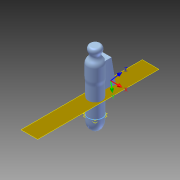
# Autodesk Inventor part: Handle_1_backup
Saved by Autodesk Inventor 2011 SP2 (Build 150309200, 309)
## iProperties
Created: 2012-02-26
Part Number: Handle_1_backup
Document SubType Name: Modeling
Designer: sungwook
Density: 1 g/cm^3
Author: sungwook
Autodesk Inventor part; units mm, degrees
note: some values were not read from the file. Chosen so that the rebuilt part matches the saved one: direction of "Hole2".
(part 1 of 18)
ref_plane "YZ Plane" through (0, 0, 0) normal (1, 0, 0) x (0, 1, 0)
sketch "Handle_0" plane through (0, 0, 0) normal (0, 0, 1) x (1, 0, 0)
  spline S0 degree 3 poles (-10017.4276, -10030.2974) (-10017.014, -10030.1564) (-10016.1737, -10029.8699) (-10014.8677, -10029.4935) (-10013.4915, -10029.1726) (-10012.0789, -10028.9345) (-10010.6777, -10028.7846) (-10009.3294, -10028.7092) (-10008.027, -10028.6839) (-10007.1723, -10028.6839) (-10006.75, -10028.6838) knots 0 0 0 0 0.131107 0.266278 0.407581 0.554823 0.69573 0.830104 0.959816 1.086502 1.086502 1.086502 1.086502
  spline S1 degree 3 poles (-10021.7321, -10032.2974) (-10021.7323, -10032.2974) (-10021.7332, -10032.2974) (-10021.7351, -10032.2974) (-10021.7383, -10032.2974) (-10021.7427, -10032.2974) (-10021.7484, -10032.2974) (-10021.7553, -10032.2974) (-10021.7635, -10032.2974) (-10021.7729, -10032.2974) (-10021.7836, -10032.2974) (-10021.7954, -10032.2974) (-10021.8085, -10032.2974) (-10021.8228, -10032.2974) (-10021.8383, -10032.2974) (-10021.8549, -10032.2974) (-10021.8727, -10032.2974) (-10021.8849, -10032.2974) (-10021.8912, -10032.2974) knots 0 0 0 0 0.003987 0.015957 0.035891 0.063749 0.099497 0.143102 0.194528 0.253743 0.320712 0.395401 0.477746 0.567575 0.664794 0.769325 0.881087 1 1 1 1
  spline S2 degree 3 poles (-10021.8912, -10032.2974) (-10021.5076, -10032.1439) (-10020.7463, -10031.8393) (-10019.2614, -10031.1643) (-10018.1607, -10030.6439) (-10017.4276, -10030.2974) knots 0 0 0 0 0.253343 0.502767 1 1 1 1
  spline S3 degree 3 poles (-10017.7909, -10013.9834) (-10017.3644, -10014.133) (-10016.4972, -10014.4372) (-10015.1487, -10014.8433) (-10013.7243, -10015.1928) (-10012.2605, -10015.4542) (-10010.8089, -10015.6192) (-10009.4142, -10015.7024) (-10008.0687, -10015.7302) (-10007.1861, -10015.7302) (-10006.75, -10015.7303) knots 0 0 0 0 0.135587 0.27568 0.422315 0.575323 0.72143 0.860365 0.994299 1.125132 1.125132 1.125132 1.125132
  line L0 (-10022.3039, -10015.9834) -> (-10006.75, -10015.9834)
  line L1 (-10006.75, -10015.7303) -> (-10006.75, -10015.9834)
  line L2 (-10006.75, -10015.9834) -> (-10006.75, -10017.9834)
  spline S4 degree 3 poles (-10006.75, -10017.9834) (-10007.6323, -10017.9834) (-10008.9768, -10017.9834) (-10010.805, -10017.9834) (-10012.253, -10017.9834) (-10013.7139, -10017.9834) (-10015.1384, -10017.9834) (-10016.4885, -10017.9834) (-10017.3635, -10017.9834) (-10017.7912, -10017.9834) knots 0 0 0 0 0.264693 0.403339 0.548464 0.699098 0.841605 0.975818 1.104119 1.104119 1.104119 1.104119
  spline S5 degree 3 poles (-10017.7912, -10017.9834) (-10018.5274, -10017.6306) (-10019.6344, -10017.1002) (-10020.9473, -10016.5195) (-10021.7151, -10016.205) (-10022.1069, -10016.0575) (-10022.3039, -10015.9834) knots 0 0 0 0 0.495968 0.745691 0.872094 1 1 1 1
  spline S6 degree 3 poles (-10022.3039, -10015.9834) (-10022.2789, -10015.9018) (-10022.229, -10015.7391) (-10022.1784, -10015.4891) (-10022.1468, -10015.237) (-10022.1364, -10014.9833) (-10022.1468, -10014.7297) (-10022.1783, -10014.4775) (-10022.2289, -10014.2276) (-10022.2788, -10014.0649) (-10022.3038, -10013.9834) knots 0 0 0 0 0.125726 0.250746 0.375528 0.500005 0.624584 0.749245 0.874433 1 1 1 1
  spline S7 degree 3 poles (-10022.3038, -10013.9834) (-10021.9144, -10013.9834) (-10021.1487, -10013.9834) (-10019.6444, -10013.9834) (-10018.5295, -10013.9834) (-10017.7909, -10013.9834) knots 0 0 0 0 0.25882 0.509015 1 1 1 1
  line L3 (-10033.25, -10030.2974) -> (-10017.4276, -10030.2974)
  line L4 (-10033.25, -10030.2974) -> (-10033.25, -10028.2974)
  line L5 (-10033.25, -10028.2974) -> (-10006.75, -10028.2974)
  line L6 (-10033.25, -10032.2974) -> (-10021.8912, -10032.2974)
  line L7 (-10033.25, -10032.2974) -> (-10033.25, -10030.2974)
  line L8 (-10033.25, -10017.9834) -> (-10017.7912, -10017.9834)
  line L9 (-10033.25, -10017.9834) -> (-10033.25, -10015.9834)
  line L10 (-10033.25, -10015.9834) -> (-10022.3039, -10015.9834)
  line L11 (-10033.25, -10015.9834) -> (-10033.25, -10013.9834)
  line L12 (-10033.25, -10013.9834) -> (-10022.3038, -10013.9834)
  line L13 (-10033.25, -10018.7294) -> (-10006.75, -10018.7294)
  line L14 (-10033.25, -10018.7294) -> (-10033.25, -10017.9834)
  line L15 (-10033.25, -10016.7294) -> (-10006.75, -10016.7294)
  line L16 (-10033.25, -10014.7294) -> (-10017.2831, -10014.7294)
  spline S8 degree 3 poles (-10006.75, -10016.3506) (-10007.1666, -10016.3506) (-10008.0095, -10016.3506) (-10009.294, -10016.3252) (-10010.6236, -10016.2493) (-10012.0057, -10016.0986) (-10013.3997, -10015.8592) (-10014.758, -10015.5367) (-10016.0468, -10015.1587) (-10016.8753, -10014.871) (-10017.2831, -10014.7294) knots 0 0 0 0 0.124973 0.252876 0.385371 0.524366 0.669742 0.809378 0.942972 1.072465 1.072465 1.072465 1.072465
  spline S9 degree 3 poles (-10022.0472, -10014.7294) (-10022.0417, -10014.8155) (-10022.0307, -10014.9878) (-10022.0416, -10015.2468) (-10022.0725, -10015.5043) (-10022.1248, -10015.7593) (-10022.1972, -10016.0104) (-10022.2891, -10016.2566) (-10022.398, -10016.4976) (-10022.4841, -10016.652) (-10022.5273, -10016.7294) knots 0 0 0 0 0.12386 0.247576 0.371585 0.495852 0.620749 0.746432 0.87277 1 1 1 1
  spline S10 degree 3 poles (-10022.5273, -10016.7294) (-10022.3413, -10016.8015) (-10021.9712, -10016.9449) (-10021.2455, -10017.2527) (-10020.357, -10017.6621) (-10019.3096, -10018.1858) (-10018.6193, -10018.548) (-10018.2736, -10018.7294) knots 0 0 0 0 0.127199 0.253182 0.502754 0.751027 1 1 1 1
  line L17 (-10035.75, -10008.8034) -> (-10035.75, -10032.8034)
  line L18 (-10149.7109, -10011.3194) -> (-10149.7109, -10030.2874)
  line L19 (-10149.3255, -10010.8327) -> (-10149.3255, -10030.7741)
  spline S11 degree 3 poles (-10130.7269, -10031.7874) (-10130.926, -10031.6416) (-10131.3276, -10031.3477) (-10132.101, -10030.7002) (-10132.8603, -10030.0211) (-10133.6568, -10029.3749) (-10134.1857, -10029.0056) (-10134.6323, -10028.7443) (-10134.9822, -10028.5682) (-10135.3467, -10028.4119) (-10135.5994, -10028.3291) (-10135.7269, -10028.2874) knots 0 0 0 0 0.074013 0.149267 0.302447 0.379596 0.456855 0.495662 0.534746 0.574288 0.614507 0.614507 0.614507 0.614507
  spline S12 degree 3 poles (-10130.7269, -10009.8194) (-10130.926, -10009.9651) (-10131.3276, -10010.2591) (-10132.101, -10010.9066) (-10132.8603, -10011.5857) (-10133.6568, -10012.2319) (-10134.1857, -10012.6012) (-10134.6323, -10012.8625) (-10134.9822, -10013.0385) (-10135.3467, -10013.1949) (-10135.5994, -10013.2777) (-10135.7269, -10013.3194) knots 0 0 0 0 0.074013 0.149267 0.302447 0.379596 0.456855 0.495662 0.534746 0.574288 0.614507 0.614507 0.614507 0.614507
  spline S13 degree 3 poles (-10125.7269, -10033.3034) (-10125.9497, -10033.3002) (-10126.3951, -10033.294) (-10127.0596, -10033.2345) (-10127.7155, -10033.1289) (-10128.3575, -10032.9694) (-10128.9818, -10032.7548) (-10129.5857, -10032.4841) (-10130.1707, -10032.1631) (-10130.5407, -10031.9132) (-10130.7269, -10031.7874) knots 0 0 0 0 0.066832 0.133581 0.19996 0.265954 0.331772 0.397749 0.464268 0.531651 0.531651 0.531651 0.531651
  spline S14 degree 3 poles (-10125.7269, -10008.3034) (-10125.9497, -10008.3065) (-10126.3951, -10008.3128) (-10127.0596, -10008.3723) (-10127.7155, -10008.4778) (-10128.3575, -10008.6374) (-10128.9818, -10008.8519) (-10129.5857, -10009.1227) (-10130.1707, -10009.4437) (-10130.5407, -10009.6936) (-10130.7269, -10009.8194) knots 0 0 0 0 0.066832 0.133581 0.19996 0.265954 0.331772 0.397749 0.464268 0.531651 0.531651 0.531651 0.531651
  arc A0 (-10149.3255, -10010.8327) -> (-10149.7109, -10011.3194) centre (-10149.2109, -10011.3194) ccw
  arc A1 (-10149.7109, -10030.2874) -> (-10149.3255, -10030.7741) centre (-10149.2109, -10030.2874) ccw
  spline S15 degree 3 poles (-10135.7269, -10028.2874) (-10135.9278, -10028.2333) (-10136.3389, -10028.1224) (-10136.9908, -10028.0381) (-10137.6833, -10028.0106) (-10138.4185, -10028.0482) (-10139.195, -10028.1445) (-10140.0117, -10028.2962) (-10140.8656, -10028.4992) (-10142.0718, -10028.8328) (-10143.63, -10029.3289) (-10145.5262, -10029.9531) (-10147.1288, -10030.4125) (-10148.3979, -10030.6807) (-10149.0212, -10030.7434) (-10149.3255, -10030.7741) knots 0 0 0 0 0.062347 0.127633 0.196641 0.270049 0.348203 0.431234 0.519115 0.611423 0.806629 1.009594 1.210352 1.306485 1.398176 1.398176 1.398176 1.398176
  spline S16 degree 3 poles (-10135.7269, -10013.3194) (-10135.9278, -10013.3735) (-10136.3389, -10013.4843) (-10136.9908, -10013.5687) (-10137.6833, -10013.5961) (-10138.4185, -10013.5586) (-10139.195, -10013.4622) (-10140.0117, -10013.3105) (-10140.8656, -10013.1076) (-10142.0718, -10012.774) (-10143.63, -10012.2779) (-10145.5262, -10011.6537) (-10147.1288, -10011.1943) (-10148.3979, -10010.9261) (-10149.0212, -10010.8633) (-10149.3255, -10010.8327) knots 0 0 0 0 0.062347 0.127633 0.196641 0.270049 0.348203 0.431234 0.519115 0.611423 0.806629 1.009594 1.210352 1.306485 1.398176 1.398176 1.398176 1.398176
  line L20 (-10150.7269, -10009.8034) -> (-10150.7269, -10031.8034)
  spline S17 degree 3 poles (-10135.7269, -10029.3034) (-10135.5108, -10029.4039) (-10135.0741, -10029.6072) (-10134.4442, -10029.9821) (-10133.8129, -10030.3902) (-10133.18, -10030.8311) (-10132.5504, -10031.3008) (-10131.7333, -10031.962) (-10131.1285, -10032.4676) (-10130.7269, -10032.8034) knots 0 0 0 0 0.071451 0.144434 0.219638 0.296973 0.375788 0.45523 0.612272 0.612272 0.612272 0.612272
  spline S18 degree 3 poles (-10135.7269, -10012.3034) (-10135.5108, -10012.2028) (-10135.0741, -10011.9996) (-10134.4442, -10011.6247) (-10133.8129, -10011.2166) (-10133.18, -10010.7757) (-10132.5504, -10010.306) (-10131.7333, -10009.6447) (-10131.1285, -10009.1391) (-10130.7269, -10008.8034) knots 0 0 0 0 0.071451 0.144434 0.219638 0.296973 0.375788 0.45523 0.612272 0.612272 0.612272 0.612272
  spline S19 degree 3 poles (-10130.7269, -10032.8034) (-10130.5423, -10032.9469) (-10130.2674, -10033.1606) (-10129.884, -10033.4163) (-10129.594, -10033.5901) (-10129.2985, -10033.7456) (-10128.9973, -10033.882) (-10128.6898, -10033.9984) (-10128.3763, -10034.0947) (-10128.0571, -10034.172) (-10127.6231, -10034.2505) (-10127.0692, -10034.306) (-10126.3992, -10034.3225) (-10125.9509, -10034.3204) (-10125.7269, -10034.3194) knots 0 0 0 0 0.070131 0.104405 0.138173 0.17151 0.20452 0.237328 0.270066 0.302853 0.33579 0.402309 0.469592 0.53679 0.53679 0.53679 0.53679
  spline S20 degree 3 poles (-10130.7269, -10008.8034) (-10130.5423, -10008.6598) (-10130.2674, -10008.4461) (-10129.884, -10008.1905) (-10129.594, -10008.0167) (-10129.2985, -10007.8612) (-10128.9973, -10007.7247) (-10128.6898, -10007.6084) (-10128.3763, -10007.5121) (-10128.0571, -10007.4348) (-10127.6231, -10007.3563) (-10127.0692, -10007.3007) (-10126.3992, -10007.2843) (-10125.9509, -10007.2864) (-10125.7269, -10007.2874) knots 0 0 0 0 0.070131 0.104405 0.138173 0.17151 0.20452 0.237328 0.270066 0.302853 0.33579 0.402309 0.469592 0.53679 0.53679 0.53679 0.53679
  spline S21 degree 3 poles (-10149.7109, -10031.8034) (-10149.3939, -10031.7865) (-10148.7265, -10031.7511) (-10147.7049, -10031.5383) (-10146.6313, -10031.2587) (-10145.1692, -10030.808) (-10143.7277, -10030.3152) (-10142.32, -10029.8454) (-10141.3329, -10029.5329) (-10140.407, -10029.2713) (-10139.5489, -10029.0697) (-10138.761, -10028.9335) (-10138.0418, -10028.87) (-10137.3871, -10028.8799) (-10136.7899, -10028.9587) (-10136.2385, -10029.099) (-10135.8958, -10029.2359) (-10135.7269, -10029.3034) knots 0 0 0 0 0.095122 0.200216 0.312183 0.428034 0.659064 0.769198 0.873257 0.96964 1.057768 1.137592 1.209313 1.274064 1.333591 1.389675 1.444205 1.444205 1.444205 1.444205
  spline S22 degree 3 poles (-10149.7109, -10009.8034) (-10149.3939, -10009.8202) (-10148.7265, -10009.8557) (-10147.7049, -10010.0685) (-10146.6313, -10010.3481) (-10145.1692, -10010.7988) (-10143.7277, -10011.2916) (-10142.32, -10011.7614) (-10141.3329, -10012.0739) (-10140.407, -10012.3355) (-10139.5489, -10012.5371) (-10138.761, -10012.6733) (-10138.0418, -10012.7368) (-10137.3871, -10012.7269) (-10136.7899, -10012.6481) (-10136.2385, -10012.5077) (-10135.8958, -10012.3709) (-10135.7269, -10012.3034) knots 0 0 0 0 0.095122 0.200216 0.312183 0.428034 0.659064 0.769198 0.873257 0.96964 1.057768 1.137592 1.209313 1.274064 1.333591 1.389675 1.444205 1.444205 1.444205 1.444205
  line L21 (-10149.7109, -10031.8034) -> (-10150.7269, -10031.8034)
  line L22 (-10149.7109, -10009.8034) -> (-10150.7269, -10009.8034)
  line L23 (-10006.75, -10012.8034) -> (-10006.75, -10015.7303)
  line L24 (-10006.75, -10017.9834) -> (-10006.75, -10028.6838)
  spline S23 degree 3 poles (-10031.75, -10033.8194) (-10030.8977, -10033.8186) (-10029.6216, -10033.8174) (-10027.9256, -10033.7166) (-10026.664, -10033.5781) (-10025.4125, -10033.368) (-10024.1727, -10033.0817) (-10022.9433, -10032.7265) (-10022.1369, -10032.4408) (-10021.7321, -10032.2974) knots 0 0 0 0 0.25561 0.382747 0.509496 0.636178 0.763224 0.891032 1.019834 1.019834 1.019834 1.019834
  spline S24 degree 3 poles (-10031.75, -10007.7874) (-10030.68, -10007.7919) (-10029.0783, -10007.7987) (-10026.9528, -10007.9822) (-10025.3776, -10008.2408) (-10023.8213, -10008.6177) (-10021.7597, -10009.2599) (-10019.25, -10010.2954) (-10016.7403, -10011.3308) (-10014.6787, -10011.973) (-10013.1224, -10012.35) (-10011.5472, -10012.6085) (-10009.4217, -10012.792) (-10007.82, -10012.7988) (-10006.75, -10012.8034) knots 0 0 0 0 0.320849 0.480281 0.639462 0.799243 0.960292 1.286737 1.613182 1.774231 1.934012 2.093192 2.252625 2.573474 2.573474 2.573474 2.573474
  line L25 (-10035.75, -10015.8034) -> (-10006.75, -10015.8034)
  line L26 (-10035.75, -10025.8034) -> (-10006.75, -10025.8034)
  line L27 (-10035.75, -10015.8404) -> (-10033.25, -10015.8404)
  line L28 (-10035.75, -10017.6184) -> (-10033.25, -10017.6184)
  line L29 (-10035.75, -10015.0944) -> (-10033.25, -10015.0944)
  line L30 (-10035.75, -10016.8724) -> (-10033.25, -10016.8724)
  line L31 (-10035.75, -10029.4084) -> (-10033.25, -10029.4084)
  line L32 (-10035.75, -10031.1864) -> (-10033.25, -10031.1864)
  line L33 (-10035.75, -10032.8034) -> (-10095.75, -10032.8034)
  line L34 (-10035.75, -10008.8034) -> (-10095.75, -10008.8034)
  line L35 (-10031.75, -10033.8194) -> (-10095.75, -10033.8194)
  line L36 (-10031.75, -10007.7874) -> (-10095.75, -10007.7874)
  spline S25 degree 3 poles (-10095.75, -10032.8034) (-10095.9588, -10032.8037) (-10096.376, -10032.8044) (-10097.0013, -10032.8424) (-10097.6226, -10032.9293) (-10098.2385, -10033.0534) (-10098.8543, -10033.1775) (-10099.4756, -10033.2644) (-10100.1009, -10033.3024) (-10100.5181, -10033.303) (-10100.7269, -10033.3034) knots 0 0 0 0 0.062631 0.12514 0.187761 0.250672 0.313584 0.376205 0.438713 0.501345 0.501345 0.501345 0.501345
  spline S26 degree 3 poles (-10095.75, -10008.8034) (-10095.9588, -10008.803) (-10096.376, -10008.8024) (-10097.0013, -10008.7644) (-10097.6226, -10008.6775) (-10098.2385, -10008.5534) (-10098.8543, -10008.4293) (-10099.4756, -10008.3424) (-10100.1009, -10008.3044) (-10100.5181, -10008.3037) (-10100.7269, -10008.3034) knots 0 0 0 0 0.062631 0.12514 0.187761 0.250672 0.313584 0.376205 0.438713 0.501345 0.501345 0.501345 0.501345
  spline S27 degree 3 poles (-10100.7269, -10034.3194) (-10100.5181, -10034.319) (-10100.1009, -10034.3184) (-10099.4756, -10034.2804) (-10098.8543, -10034.1935) (-10098.2385, -10034.0694) (-10097.6226, -10033.9453) (-10097.0013, -10033.8584) (-10096.376, -10033.8204) (-10095.9588, -10033.8197) (-10095.75, -10033.8194) knots 0 0 0 0 0.062631 0.12514 0.187761 0.250672 0.313584 0.376205 0.438713 0.501345 0.501345 0.501345 0.501345
  spline S28 degree 3 poles (-10100.7269, -10007.2874) (-10100.5181, -10007.2877) (-10100.1009, -10007.2884) (-10099.4756, -10007.3264) (-10098.8543, -10007.4133) (-10098.2385, -10007.5374) (-10097.6226, -10007.6615) (-10097.0013, -10007.7484) (-10096.376, -10007.7864) (-10095.9588, -10007.787) (-10095.75, -10007.7874) knots 0 0 0 0 0.062631 0.12514 0.187761 0.250672 0.313584 0.376205 0.438713 0.501345 0.501345 0.501345 0.501345
  line L37 (-10100.7269, -10033.3034) -> (-10125.7269, -10033.3034)
  line L38 (-10100.7269, -10008.3034) -> (-10125.7269, -10008.3034)
  line L39 (-10100.7269, -10034.3194) -> (-10125.7269, -10034.3194)
  line L40 (-10100.7269, -10007.2874) -> (-10125.7269, -10007.2874)
  point P0 (-10079.453, -10020.7457)
  point P1 (-10016.1834, -10029.8841)
  point P2 (-10014.8845, -10029.5102)
  point P3 (-10013.5079, -10029.1911)
  point P4 (-10012.056, -10028.946)
  point P5 (-10010.6551, -10028.7944)
  point P6 (-10009.3137, -10028.7166)
  point P7 (-10008.0169, -10028.6879)
  point P8 (-10021.7328, -10032.2974)
  point P9 (-10021.7347, -10032.2974)
  point P10 (-10021.7378, -10032.2974)
  point P11 (-10021.7423, -10032.2974)
  point P12 (-10021.748, -10032.2974)
  point P13 (-10021.7549, -10032.2974)
  point P14 (-10021.7631, -10032.2974)
  point P15 (-10021.7725, -10032.2974)
  point P16 (-10021.7831, -10032.2974)
  point P17 (-10021.795, -10032.2974)
  point P18 (-10021.8081, -10032.2974)
  point P19 (-10021.8224, -10032.2974)
  point P20 (-10021.8379, -10032.2974)
  point P21 (-10021.8545, -10032.2974)
  point P22 (-10021.8723, -10032.2974)
  point P23 (-10020.7441, -10031.8281)
  point P24 (-10019.6303, -10031.3297)
  point P25 (-10016.5082, -10014.4228)
  point P26 (-10015.1664, -10014.8256)
  point P27 (-10013.7418, -10015.1728)
  point P28 (-10012.2355, -10015.4418)
  point P29 (-10010.784, -10015.6086)
  point P30 (-10009.3973, -10015.6942)
  point P31 (-10008.0583, -10015.7258)
  point P32 (-10009.3969, -10017.9834)
  point P33 (-10010.7834, -10017.9834)
  point P34 (-10012.2346, -10017.9834)
  point P35 (-10013.741, -10017.9834)
  point P36 (-10015.166, -10017.9834)
  point P37 (-10016.5082, -10017.9834)
  point P38 (-10020.0068, -10016.9401)
  point P39 (-10021.1359, -10016.4444)
  point P40 (-10021.7139, -10016.2087)
  point P41 (-10022.2329, -10015.7376)
  point P42 (-10022.1815, -10015.4884)
  point P43 (-10022.1503, -10015.2365)
  point P44 (-10022.1399, -10014.9834)
  point P45 (-10022.1503, -10014.7301)
  point P46 (-10022.1814, -10014.4784)
  point P47 (-10022.2329, -10014.2289)
  point P48 (-10021.1357, -10013.9834)
  point P49 (-10020.0066, -10013.9834)
  point P50 (-10007.9997, -10016.3465)
  point P51 (-10009.2784, -10016.3177)
  point P52 (-10010.6011, -10016.2395)
  point P53 (-10011.9826, -10016.0871)
  point P54 (-10013.4154, -10015.8407)
  point P55 (-10014.7744, -10015.5201)
  point P56 (-10016.0564, -10015.1444)
  point P57 (-10022.0353, -10014.988)
  point P58 (-10022.0449, -10015.2463)
  point P59 (-10022.076, -10015.5036)
  point P60 (-10022.128, -10015.758)
  point P61 (-10022.2002, -10016.0089)
  point P62 (-10022.2917, -10016.2551)
  point P63 (-10022.4011, -10016.4954)
  point P64 (-10021.9706, -10016.9485)
  point P65 (-10021.4247, -10017.1789)
  point P66 (-10020.3579, -10017.6686)
  point P67 (-10019.3124, -10018.1887)
  point P68 (-10131.3194, -10031.3438)
  point P69 (-10131.8999, -10030.865)
  point P70 (-10133.0599, -10029.8645)
  point P71 (-10133.6622, -10029.3824)
  point P72 (-10134.2982, -10028.9438)
  point P73 (-10134.6335, -10028.7483)
  point P74 (-10134.9825, -10028.5725)
  point P75 (-10135.3466, -10028.4182)
  point P76 (-10131.3194, -10010.2629)
  point P77 (-10131.8999, -10010.7418)
  point P78 (-10133.0599, -10011.7423)
  point P79 (-10133.6622, -10012.2243)
  point P80 (-10134.2982, -10012.663)
  point P81 (-10134.6335, -10012.8584)
  point P82 (-10134.9825, -10013.0343)
  point P83 (-10135.3466, -10013.1886)
  point P84 (-10126.395, -10033.2856)
  point P85 (-10127.0599, -10033.2266)
  point P86 (-10127.715, -10033.1196)
  point P87 (-10128.3553, -10032.96)
  point P88 (-10128.9777, -10032.7458)
  point P89 (-10129.5802, -10032.4769)
  point P90 (-10130.1628, -10032.1559)
  point P91 (-10126.395, -10008.3212)
  point P92 (-10127.0599, -10008.3802)
  point P93 (-10127.715, -10008.4872)
  point P94 (-10128.3553, -10008.6468)
  point P95 (-10128.9777, -10008.861)
  point P96 (-10129.5802, -10009.1299)
  point P97 (-10130.1628, -10009.4509)
  point P98 (-10136.3323, -10028.1384)
  point P99 (-10136.979, -10028.0491)
  point P100 (-10137.6686, -10028.0213)
  point P101 (-10138.4018, -10028.0559)
  point P102 (-10139.1777, -10028.1501)
  point P103 (-10139.9944, -10028.2998)
  point P104 (-10140.8499, -10028.5008)
  point P105 (-10141.7401, -10028.745)
  point P106 (-10143.6043, -10029.324)
  point P107 (-10145.5373, -10029.9428)
  point P108 (-10147.4723, -10030.4776)
  point P109 (-10148.415, -10030.6662)
  point P110 (-10136.3323, -10013.4684)
  point P111 (-10136.979, -10013.5577)
  point P112 (-10137.6686, -10013.5854)
  point P113 (-10138.4018, -10013.5508)
  point P114 (-10139.1777, -10013.4567)
  point P115 (-10139.9944, -10013.307)
  point P116 (-10140.8499, -10013.106)
  point P117 (-10141.7401, -10012.8618)
  point P118 (-10143.6043, -10012.2828)
  point P119 (-10145.5373, -10011.6639)
  point P120 (-10147.4723, -10011.1292)
  point P121 (-10148.415, -10010.9405)
  point P122 (-10135.0842, -10029.6156)
  point P123 (-10134.453, -10029.982)
  point P124 (-10133.8212, -10030.3899)
  point P125 (-10133.1864, -10030.8316)
  point P126 (-10132.5552, -10031.3036)
  point P127 (-10131.9353, -10031.8004)
  point P128 (-10135.0842, -10011.9912)
  point P129 (-10134.453, -10011.6248)
  point P130 (-10133.8212, -10011.2169)
  point P131 (-10133.1864, -10010.7751)
  point P132 (-10132.5552, -10010.3032)
  point P133 (-10131.9353, -10009.8064)
  point P134 (-10130.1663, -10033.2248)
  point P135 (-10129.8811, -10033.4149)
  point P136 (-10129.5913, -10033.5881)
  point P137 (-10129.2961, -10033.7431)
  point P138 (-10128.9953, -10033.8791)
  point P139 (-10128.6885, -10033.9952)
  point P140 (-10128.3756, -10034.0915)
  point P141 (-10128.0569, -10034.1687)
  point P142 (-10127.7329, -10034.2277)
  point P143 (-10127.0714, -10034.2975)
  point P144 (-10126.3989, -10034.3192)
  point P145 (-10130.1663, -10008.382)
  point P146 (-10129.8811, -10008.1919)
  point P147 (-10129.5913, -10008.0187)
  point P148 (-10129.2961, -10007.8636)
  point P149 (-10128.9953, -10007.7277)
  point P150 (-10128.6885, -10007.6116)
  point P151 (-10128.3756, -10007.5153)
  point P152 (-10128.0569, -10007.4381)
  point P153 (-10127.7329, -10007.3791)
  point P154 (-10127.0714, -10007.3093)
  point P155 (-10126.3989, -10007.2876)
  point P156 (-10148.7625, -10031.7301)
  point P157 (-10147.7298, -10031.5349)
  point P158 (-10146.646, -10031.2541)
  point P159 (-10145.5375, -10030.9174)
  point P160 (-10143.3452, -10030.1884)
  point P161 (-10142.2998, -10029.8418)
  point P162 (-10141.3069, -10029.5306)
  point P163 (-10140.3786, -10029.2711)
  point P164 (-10139.52, -10029.0723)
  point P165 (-10138.7328, -10028.9404)
  point P166 (-10138.018, -10028.8809)
  point P167 (-10137.3706, -10028.8932)
  point P168 (-10136.7806, -10028.9721)
  point P169 (-10136.2375, -10029.1121)
  point P170 (-10148.7625, -10009.8767)
  point P171 (-10147.7298, -10010.0718)
  point P172 (-10146.646, -10010.3527)
  point P173 (-10145.5375, -10010.6894)
  point P174 (-10143.3452, -10011.4183)
  point P175 (-10142.2998, -10011.765)
  point P176 (-10141.3069, -10012.0762)
  point P177 (-10140.3786, -10012.3357)
  point P178 (-10139.52, -10012.5344)
  point P179 (-10138.7328, -10012.6663)
  point P180 (-10138.018, -10012.7259)
  point P181 (-10137.3706, -10012.7136)
  point P182 (-10136.7806, -10012.6347)
  point P183 (-10136.2375, -10012.4947)
  point P184 (-10029.1941, -10033.7838)
  point P185 (-10027.9252, -10033.706)
  point P186 (-10026.6654, -10033.5662)
  point P187 (-10025.4162, -10033.3557)
  point P188 (-10024.178, -10033.0712)
  point P189 (-10022.9504, -10032.7155)
  point P190 (-10028.5423, -10007.8595)
  point P191 (-10026.9544, -10008.0025)
  point P192 (-10025.3836, -10008.2599)
  point P193 (-10023.83, -10008.6332)
  point P194 (-10022.2919, -10009.1107)
  point P195 (-10019.25, -10010.2954)
  point P196 (-10016.2081, -10011.48)
  point P197 (-10014.67, -10011.9576)
  point P198 (-10013.1164, -10012.3309)
  point P199 (-10011.5456, -10012.5882)
  dimension "d16" = 25
  dimension "d17" = 17
  dimension "d18" = 10
  dimension "d19" = 24
  dimension "d20" = 5
  dimension "d22" = 1.016
  dimension "d23" = 1.016
  dimension "d25" = 2
  dimension "d26" = 20
  dimension "d27" = 0.762
  dimension "d28" = 13
  dimension "d91" = 11
  dimension "d92" = 2
sketch "Top" plane through (0, 0, 0) normal (0, 0, 1) x (1, 0, 0)
  line L0 (-10061.3845, -10012.5621) -> (-10061.3896, -10012.5375)
  ellipse E0 centre (-10061.4073, -10012.4391) end of major axis (-10061.568, -10011.6553) minor radius 0.0024 (-10061.4418, -10012.2826) -> (-10061.3896, -10012.5375) ccw
  ellipse E1 centre (-10061.4073, -10012.4391) end of major axis (-10061.568, -10011.6553) minor radius 0.0024 (-10061.568, -10011.6553) -> (-10061.4775, -10012.1074) ccw
  line L1 (-10061.5673, -10011.6552) -> (-10061.568, -10011.6553)
  ellipse E2 centre (-10061.4073, -10025.7549) end of major axis (-10061.568, -10026.5386) minor radius 0.0024 (-10061.4778, -10026.0879) -> (-10061.568, -10026.5386) ccw
  line L2 (-10061.2026, -10024.7419) -> (-10061.1551, -10024.5095)
  line L3 (-10061.5673, -10026.5388) -> (-10061.568, -10026.5386)
  ellipse E3 centre (-10061.2636, -10012.9714) end of major axis (-10061.5191, -10012.2133) minor radius 0.0023 (-10061.2891, -10012.903) -> (-10061.2381, -10013.0544) ccw
  ellipse E4 centre (-10061.2636, -10012.9714) end of major axis (-10061.5191, -10012.2133) minor radius 0.0023 (-10061.3289, -10012.7848) -> (-10061.2911, -10012.8971) ccw
  ellipse E5 centre (-10061.2636, -10012.9714) end of major axis (-10061.5191, -10012.2133) minor radius 0.0023 (-10061.5191, -10012.2133) -> (-10061.4629, -10012.3848) ccw
  line L4 (-10061.511, -10012.2106) -> (-10061.5191, -10012.2133)
  line L5 (-10061.4095, -10014.7699) -> (-10066.3154, -10016.4234)
  ellipse E6 centre (-10060.3502, -10010.3291) end of major axis (-10060.1614, -10011.1065) minor radius 0.1369 (-10060.4111, -10010.6238) -> (-10060.4058, -10010.6409) ccw
  line L6 (-10060.339, -10010.9116) -> (-10060.3893, -10010.721)
  ellipse E7 centre (-10059.3928, -10010.0966) end of major axis (-10059.2748, -10010.5825) minor radius 0.0856 (-10059.4497, -10010.217) -> (-10059.2564, -10010.3635) ccw
  ellipse E8 centre (-10061.434, -10028.7875) end of major axis (-10061.4139, -10029.5872) minor radius 0.1339 (-10061.5458, -10029.1388) -> (-10061.4139, -10029.5872) ccw
  line L7 (-10061.5672, -10028.8146) -> (-10061.6147, -10027.2411)
  line L8 (-10061.6147, -10027.2411) -> (-10061.4173, -10027.2361)
  ellipse E9 centre (-10059.4629, -10028.7378) end of major axis (-10059.4427, -10029.5376) minor radius 0.1339 (-10059.5955, -10028.4658) -> (-10059.5961, -10028.7649) ccw
  line L9 (-10061.6147, -10027.2411) -> (-10062.0082, -10027.251)
  line L10 (-10062.6831, -10027.268) -> (-10063.6487, -10027.2923)
  ellipse E10 centre (-10075.1335, -10029.1327) end of major axis (-10075.0809, -10031.222) minor radius 0.3499 (-10075.432, -10029.9867) -> (-10075.403, -10030.2415) ccw
  ellipse E11 centre (-10074.2465, -10029.1103) end of major axis (-10074.1938, -10031.1997) minor radius 0.3499 (-10074.5441, -10029.973) -> (-10074.5173, -10030.2086) ccw
  ellipse E12 centre (-10074.2465, -10029.1103) end of major axis (-10074.2087, -10030.6098) minor radius 0.2511 (-10074.479, -10028.3167) -> (-10074.1506, -10030.5661) ccw
  ellipse E13 centre (-10059.4629, -10028.7378) end of major axis (-10059.4503, -10029.2377) minor radius 0.0837 (-10059.5439, -10028.8115) -> (-10059.3841, -10028.9863) ccw
  ellipse E14 centre (-10061.4873, -10026.3357) end of major axis (-10061.5444, -10027.1336) minor radius 0.0023 (-10061.4978, -10026.4498) -> (-10061.5444, -10027.1336) ccw
  line L11 (-10061.4978, -10026.4498) -> (-10061.4936, -10026.3911)
  line L12 (-10061.4768, -10026.1545) -> (-10061.3871, -10024.8951)
  line L13 (-10061.3871, -10024.8951) -> (-10061.1735, -10024.9104)
  line L14 (-10061.5312, -10027.1346) -> (-10061.5444, -10027.1336)
  line L15 (-10061.3871, -10024.8951) -> (-10063.0521, -10024.7759)
  line L16 (-10061.8223, -10012.9757) -> (-10061.4801, -10012.9079)
  line L17 (-10060.9987, -10013.9439) -> (-10061.2701, -10012.4706)
  ellipse E15 centre (-10061.3812, -10012.4032) end of major axis (-10061.5366, -10011.6185) minor radius 0.0964 (-10061.2701, -10012.4706) -> (-10061.5629, -10011.7613) ccw
  line L18 (-10061.5629, -10011.7613) -> (-10061.554, -10012.2831)
  line L19 (-10061.5288, -10011.6169) -> (-10061.5366, -10011.6185)
  line L20 (-10061.7043, -10010.4615) -> (-10061.6005, -10010.4506)
  line L21 (-10061.3966, -10010.9672) -> (-10061.4932, -10010.0915)
  ellipse E16 centre (-10061.4703, -10009.985) end of major axis (-10061.5536, -10009.1894) minor radius 0.0342 (-10061.5599, -10009.2247) -> (-10061.4932, -10010.0915) ccw
  ellipse E17 centre (-10075.2821, -10011.4314) end of major axis (-10075.4997, -10009.3527) minor radius 0.0893 (-10075.5171, -10009.4951) -> (-10075.497, -10009.9963) ccw
  ellipse E18 centre (-10074.3878, -10011.3377) end of major axis (-10074.6054, -10009.2591) minor radius 0.0893 (-10074.6228, -10009.4041) -> (-10074.6224, -10009.4715) ccw
  ellipse E19 centre (-10059.483, -10009.7769) end of major axis (-10059.4309, -10010.2742) minor radius 0.0214 (-10059.4577, -10010.1534) -> (-10059.44, -10010.2508) ccw
  ellipse E20 centre (-10059.483, -10009.7769) end of major axis (-10059.535, -10009.2797) minor radius 0.0214 (-10059.5392, -10009.3196) -> (-10059.5225, -10009.5891) ccw
  ellipse E21 centre (-10060.1471, -10022.397) end of major axis (-10060.0012, -10021.6908) minor radius 0.4312 (-10060.1977, -10023.1053) -> (-10060.1347, -10023.0885) ccw
  line L22 (-10062.0925, -10026.7931) -> (-10061.5327, -10026.8517)
  ellipse E22 centre (-10061.4703, -10028.2089) end of major axis (-10061.387, -10027.4133) minor radius 0.0342 (-10061.5078, -10028.2395) -> (-10061.5603, -10028.9423) ccw
  line L23 (-10061.5078, -10028.2395) -> (-10061.4036, -10027.2264)
  line L24 (-10061.5167, -10026.6566) -> (-10062.0819, -10026.5974)
  ellipse E23 centre (-10075.2821, -10026.7626) end of major axis (-10075.4997, -10028.8412) minor radius 0.0893 (-10075.497, -10028.1977) -> (-10075.5171, -10028.6989) ccw
  ellipse E24 centre (-10074.3878, -10026.8563) end of major axis (-10074.6054, -10028.9349) minor radius 0.0893 (-10074.6224, -10028.7225) -> (-10074.6228, -10028.7899) ccw
  ellipse E25 centre (-10074.3878, -10026.8563) end of major axis (-10074.544, -10028.3481) minor radius 0.0641 (-10074.5544, -10028.3079) -> (-10074.5256, -10028.3112) ccw
  ellipse E26 centre (-10059.483, -10028.417) end of major axis (-10059.4309, -10027.9198) minor radius 0.0214 (-10059.4268, -10027.9506) -> (-10059.4577, -10028.0406) ccw
  ellipse E27 centre (-10059.483, -10028.417) end of major axis (-10059.535, -10028.9143) minor radius 0.0214 (-10059.5225, -10028.6049) -> (-10059.5242, -10028.883) ccw
  line L25 (-10064.1249, -10023.9215) -> (-10061.096, -10024.5212)
  line L26 (-10061.5488, -10026.2255) -> (-10061.5556, -10026.3034)
  ellipse E28 centre (-10061.3812, -10025.7908) end of major axis (-10061.5366, -10026.5755) minor radius 0.0964 (-10061.5556, -10026.3034) -> (-10061.3085, -10025.9158) ccw
  line L27 (-10061.3085, -10025.9158) -> (-10060.9802, -10024.3902)
  line L28 (-10060.9802, -10024.3902) -> (-10060.9339, -10024.3993)
  line L29 (-10061.5288, -10026.5771) -> (-10061.5366, -10026.5755)
  line L30 (-10061.0155, -10024.4456) -> (-10060.9802, -10024.3902)
  line L31 (-10060.9802, -10024.3902) -> (-10064.1073, -10023.771)
  line L32 (-10061.4717, -10012.1079) -> (-10061.4838, -10011.9398)
  ellipse E29 centre (-10061.4873, -10011.8583) end of major axis (-10061.5444, -10011.0604) minor radius 0.0023 (-10061.5444, -10011.0604) -> (-10061.4838, -10011.9398) ccw
  line L33 (-10061.5312, -10011.0594) -> (-10061.5444, -10011.0604)
  line L34 (-10064.1804, -10013.7036) -> (-10064.1912, -10013.7044)
  line L35 (-10061.7739, -10009.83) -> (-10061.5814, -10009.8348)
  line L36 (-10061.5711, -10011.0479) -> (-10061.5694, -10009.5171)
  ellipse E30 centre (-10061.434, -10009.4065) end of major axis (-10061.4139, -10008.6067) minor radius 0.1339 (-10061.4139, -10008.6067) -> (-10061.5694, -10009.5171) ccw
  ellipse E31 centre (-10075.1335, -10009.0613) end of major axis (-10075.1862, -10011.1506) minor radius 0.3499 (-10075.403, -10007.9525) -> (-10075.432, -10008.2073) ccw
  ellipse E32 centre (-10074.2465, -10009.0837) end of major axis (-10074.2991, -10011.173) minor radius 0.3499 (-10074.5173, -10007.9854) -> (-10074.5441, -10008.2209) ccw
  ellipse E33 centre (-10074.2465, -10009.0837) end of major axis (-10074.2087, -10007.5841) minor radius 0.2511 (-10074.1388, -10007.648) -> (-10074.479, -10009.8773) ccw
  ellipse E34 centre (-10060.4484, -10009.4313) end of major axis (-10060.4686, -10010.2311) minor radius 0.1339 (-10060.5838, -10009.542) -> (-10060.5838, -10009.562) ccw
  ellipse E35 centre (-10059.4629, -10009.4562) end of major axis (-10059.4755, -10009.956) minor radius 0.0837 (-10059.3841, -10009.2077) -> (-10059.3859, -10009.1845) ccw
  ellipse E36 centre (-10059.4629, -10009.4562) end of major axis (-10059.4503, -10008.9563) minor radius 0.0837 (-10059.5185, -10009.1313) -> (-10059.5439, -10009.3824) ccw
  line L37 (-10060.382, -10027.3959) -> (-10060.3554, -10027.2815)
  ellipse E37 centre (-10060.3502, -10027.8649) end of major axis (-10060.539, -10028.6423) minor radius 0.1369 (-10060.4058, -10027.5531) -> (-10060.4116, -10027.5717) ccw
  ellipse E38 centre (-10059.3928, -10028.0974) end of major axis (-10059.2748, -10027.6115) minor radius 0.0856 (-10059.2564, -10027.8305) -> (-10059.4497, -10027.977) ccw
  ellipse E39 centre (-10061.2636, -10025.2226) end of major axis (-10061.5191, -10025.9807) minor radius 0.0023 (-10061.4633, -10025.8105) -> (-10061.5191, -10025.9807) ccw
  line L38 (-10060.3126, -10024.003) -> (-10059.8526, -10024.158)
  line L39 (-10061.511, -10025.9834) -> (-10061.5191, -10025.9807)
  line L40 (-10062.9976, -10023.098) -> (-10066.6582, -10021.8643)
  line L41 (-10059.9783, -10023.9188) -> (-10059.8526, -10024.158)
  line L42 (-10059.8526, -10024.158) -> (-10059.8602, -10024.1814)
  line L43 (-10059.9613, -10024.4811) -> (-10059.8526, -10024.158)
  line L44 (-10061.3433, -10012.7426) -> (-10061.3778, -10012.5868)
  ellipse E40 centre (-10061.3928, -10012.5071) end of major axis (-10061.5656, -10011.726) minor radius 0.0026 (-10061.4062, -10012.4585) -> (-10061.3778, -10012.5868) ccw
  ellipse E41 centre (-10061.3928, -10012.5071) end of major axis (-10061.5656, -10011.726) minor radius 0.0026 (-10061.4319, -10012.3422) -> (-10061.4069, -10012.4554) ccw
  ellipse E42 centre (-10061.3928, -10012.5071) end of major axis (-10061.5656, -10011.726) minor radius 0.0026 (-10061.5656, -10011.726) -> (-10061.4756, -10012.1433) ccw
  line L45 (-10061.5636, -10011.7255) -> (-10061.5656, -10011.726)
  ellipse E43 centre (-10059.3459, -10009.7776) end of major axis (-10059.4343, -10008.9825) minor radius 0.2631 (-10059.1442, -10010.4641) -> (-10059.0982, -10010.3179) ccw
  ellipse E44 centre (-10059.3459, -10009.7776) end of major axis (-10059.4343, -10008.9825) minor radius 0.2631 (-10059.214, -10009.2163) -> (-10059.3095, -10009.0518) ccw
  ellipse E45 centre (-10059.3459, -10028.4163) end of major axis (-10059.4343, -10029.2114) minor radius 0.2631 (-10059.5958, -10028.9456) -> (-10059.5505, -10029.0966) ccw
  ellipse E46 centre (-10059.3459, -10028.4163) end of major axis (-10059.4343, -10029.2114) minor radius 0.2631 (-10059.5353, -10029.1269) -> (-10059.5301, -10029.1359) ccw
  ellipse E47 centre (-10059.3459, -10028.4163) end of major axis (-10059.4343, -10029.2114) minor radius 0.2631 (-10059.383, -10029.2025) -> (-10059.214, -10028.9777) ccw
  ellipse E48 centre (-10059.3459, -10028.4163) end of major axis (-10059.2575, -10027.6212) minor radius 0.2631 (-10059.0982, -10027.8761) -> (-10059.1442, -10027.7299) ccw
  line L46 (-10060.6032, -10014.6914) -> (-10060.6494, -10014.5724)
  ellipse E49 centre (-10061.1947, -10013.1618) end of major axis (-10061.4841, -10012.416) minor radius 0.0025 (-10061.2445, -10013.0401) -> (-10061.2381, -10013.0566) ccw
  ellipse E50 centre (-10061.1947, -10013.1618) end of major axis (-10061.4841, -10012.416) minor radius 0.0025 (-10061.281, -10012.9458) -> (-10061.2623, -10012.9942) ccw
  ellipse E51 centre (-10061.1947, -10013.1618) end of major axis (-10061.4841, -10012.416) minor radius 0.0025 (-10061.4841, -10012.416) -> (-10061.4575, -10012.4875) ccw
  line L47 (-10059.671, -10014.3296) -> (-10060.6032, -10014.6914)
  ellipse E52 centre (-10059.3301, -10012.4382) end of major axis (-10059.0407, -10013.184) minor radius 0.0025 (-10059.2158, -10012.7391) -> (-10059.215, -10012.7287) ccw
  line L48 (-10059.0407, -10013.184) -> (-10059.973, -10013.5458)
  line L49 (-10061.4689, -10012.4101) -> (-10061.4841, -10012.416)
  line L50 (-10060.6032, -10014.6914) -> (-10065.5823, -10016.6237)
  line L51 (-10059.9707, -10013.5449) -> (-10059.671, -10014.3296)
  line L52 (-10059.671, -10014.3296) -> (-10059.8563, -10014.6799)
  ellipse E53 centre (-10059.9815, -10014.3522) end of major axis (-10060.3662, -10015.2269) minor radius 0.2554 (-10060.2929, -10015.2239) -> (-10059.8563, -10014.6799) ccw
  line L53 (-10060.2929, -10015.2239) -> (-10064.1601, -10016.7247)
  ellipse E54 centre (-10060.2624, -10012.8) end of major axis (-10059.973, -10013.5458) minor radius 0.0025 (-10060.0313, -10013.3994) -> (-10059.973, -10013.5458) ccw
  line L54 (-10059.671, -10014.3296) -> (-10060.0304, -10013.4041)
  ellipse E55 centre (-10059.3301, -10012.4382) end of major axis (-10059.1492, -10012.9043) minor radius 0.0015 (-10059.2156, -10012.7366) -> (-10059.2152, -10012.7312) ccw
  ellipse E56 centre (-10060.3058, -10010.4683) end of major axis (-10060.0841, -10011.237) minor radius 0.1461 (-10060.3936, -10010.678) -> (-10060.3074, -10010.9099) ccw
  line L55 (-10060.3246, -10010.9108) -> (-10060.3929, -10010.6857)
  ellipse E57 centre (-10059.3611, -10010.1959) end of major axis (-10059.2226, -10010.6764) minor radius 0.0913 (-10059.4494, -10010.2192) -> (-10059.2273, -10010.3551) ccw
  ellipse E58 centre (-10059.3611, -10010.1959) end of major axis (-10059.1395, -10010.9646) minor radius 0.1461 (-10059.4076, -10010.5231) -> (-10059.1442, -10010.4641) ccw
  line L56 (-10059.1395, -10010.9646) -> (-10059.5247, -10011.0757)
  line L57 (-10062.35, -10018.4914) -> (-10062.8067, -10018.5197)
  line L58 (-10059.925, -10023.5766) -> (-10059.7889, -10023.4993)
  line L59 (-10059.7889, -10023.4993) -> (-10059.8958, -10023.0225)
  ellipse E59 centre (-10059.3774, -10021.7447) end of major axis (-10059.1723, -10022.518) minor radius 0.1421 (-10059.1723, -10022.518) -> (-10059.1558, -10022.1003) ccw
  line L60 (-10059.1723, -10022.518) -> (-10059.8325, -10022.6931)
  line L61 (-10061.5938, -10028.2973) -> (-10061.7671, -10028.3061)
  line L62 (-10061.6914, -10027.55) -> (-10061.6309, -10027.5469)
  ellipse E60 centre (-10061.4209, -10028.899) end of major axis (-10061.3805, -10029.698) minor radius 0.143 (-10061.5409, -10029.1817) -> (-10061.3805, -10029.698) ccw
  line L63 (-10061.5639, -10028.9014) -> (-10061.6417, -10027.3285)
  line L64 (-10061.6417, -10027.3285) -> (-10061.6121, -10027.327)
  ellipse E61 centre (-10059.4556, -10028.7997) end of major axis (-10059.4152, -10029.5986) minor radius 0.143 (-10059.5711, -10029.1195) -> (-10059.3095, -10029.1422) ccw
  ellipse E62 centre (-10059.4556, -10028.7997) end of major axis (-10059.4152, -10029.5986) minor radius 0.143 (-10059.6035, -10028.5289) -> (-10059.5986, -10028.8021) ccw
  line L65 (-10059.4152, -10029.5986) -> (-10061.3805, -10029.698)
  line L66 (-10061.6417, -10027.3285) -> (-10061.6768, -10027.3303)
  line L67 (-10062.6995, -10027.382) -> (-10063.5205, -10027.4235)
  line L68 (-10061.583, -10028.5157) -> (-10061.7936, -10028.5263)
  ellipse E63 centre (-10075.0796, -10029.5896) end of major axis (-10074.9741, -10031.6769) minor radius 0.3735 (-10075.403, -10030.2415) -> (-10074.9741, -10031.6769) ccw
  ellipse E64 centre (-10074.1952, -10029.5449) end of major axis (-10074.0897, -10031.6322) minor radius 0.3735 (-10074.5173, -10030.2086) -> (-10073.8826, -10031.1795) ccw
  line L69 (-10074.9741, -10031.6769) -> (-10074.0897, -10031.6322)
  ellipse E65 centre (-10074.1952, -10029.5449) end of major axis (-10074.1195, -10031.0429) minor radius 0.2681 (-10074.4107, -10028.3246) -> (-10074.0103, -10030.8872) ccw
  ellipse E66 centre (-10059.4556, -10028.7997) end of major axis (-10059.4303, -10029.299) minor radius 0.0894 (-10059.5442, -10028.8152) -> (-10059.3634, -10028.9852) ccw
  line L70 (-10061.5129, -10025.662) -> (-10061.943, -10025.6394)
  line L71 (-10063.0799, -10025.0236) -> (-10062.8856, -10025.0339)
  line L72 (-10061.8722, -10025.0871) -> (-10061.4268, -10025.1105)
  ellipse E67 centre (-10061.4926, -10026.4207) end of major axis (-10061.5345, -10027.2196) minor radius 0.0026 (-10061.4999, -10026.5116) -> (-10061.5345, -10027.2196) ccw
  line L73 (-10061.4999, -10026.5116) -> (-10061.4184, -10024.9491)
  line L74 (-10061.4184, -10024.9491) -> (-10061.3911, -10024.9506)
  ellipse E68 centre (-10059.4953, -10026.5256) end of major axis (-10059.5373, -10027.3245) minor radius 0.0026 (-10059.5154, -10026.8628) -> (-10059.5102, -10026.8534) ccw
  line L75 (-10059.5373, -10027.3245) -> (-10061.5345, -10027.2196)
  line L76 (-10061.4184, -10024.9491) -> (-10063.0597, -10024.8629)
  line L77 (-10061.5231, -10025.8233) -> (-10061.7585, -10025.8109)
  ellipse E69 centre (-10059.4953, -10026.5256) end of major axis (-10059.5216, -10027.0249) minor radius 0.0016 (-10059.5141, -10026.8605) -> (-10059.5115, -10026.8557) ccw
  line L78 (-10061.5002, -10013.9011) -> (-10064.1038, -10014.4529)
  ellipse E70 centre (-10061.3509, -10012.4578) end of major axis (-10061.6412, -10011.0883) minor radius 0.2113 (-10061.4355, -10013.0055) -> (-10061.4289, -10013.0293) ccw
  line L79 (-10061.7995, -10013.0826) -> (-10061.4355, -10013.0055)
  line L80 (-10060.9127, -10014.0333) -> (-10060.9618, -10013.9367)
  line L81 (-10061.4355, -10013.0055) -> (-10061.4744, -10012.9289)
  line L82 (-10060.9127, -10014.0333) -> (-10061.2203, -10012.4934)
  ellipse E71 centre (-10061.3509, -10012.4578) end of major axis (-10061.5168, -10011.6752) minor radius 0.1207 (-10061.2203, -10012.4934) -> (-10061.5545, -10011.8363) ccw
  line L83 (-10061.5545, -10011.8363) -> (-10061.5534, -10012.7525)
  line L84 (-10059.9457, -10013.8283) -> (-10060.9127, -10014.0333)
  ellipse E72 centre (-10059.4168, -10012.0479) end of major axis (-10059.2509, -10012.8305) minor radius 0.1207 (-10059.2158, -10012.7391) -> (-10059.5154, -10011.3312) ccw
  line L85 (-10061.5089, -10011.6736) -> (-10061.5168, -10011.6752)
  line L86 (-10060.9127, -10014.0333) -> (-10064.0792, -10014.7044)
  line L87 (-10059.9457, -10013.8283) -> (-10060.2034, -10014.1501)
  ellipse E73 centre (-10060.3647, -10013.8329) end of major axis (-10060.93, -10014.6265) minor radius 0.32 (-10060.8092, -10014.6427) -> (-10060.2034, -10014.1501) ccw
  line L88 (-10060.8092, -10014.6427) -> (-10067.07, -10015.9697)
  line L89 (-10059.9457, -10013.8283) -> (-10060.2532, -10012.2885)
  line L90 (-10061.5263, -10011.4206) -> (-10062.088, -10011.4839)
  line L91 (-10061.6958, -10010.5467) -> (-10061.6031, -10010.5362)
  line L92 (-10061.3782, -10010.9662) -> (-10061.478, -10010.0971)
  ellipse E74 centre (-10061.4695, -10010.0209) end of major axis (-10061.5591, -10009.226) minor radius 0.017 (-10061.5607, -10009.2386) -> (-10061.478, -10010.0971) ccw
  ellipse E75 centre (-10059.4825, -10009.7968) end of major axis (-10059.3929, -10010.5918) minor radius 0.017 (-10059.5711, -10009.0745) -> (-10059.4076, -10010.5231) ccw
  line L93 (-10061.567, -10011.6851) -> (-10062.0742, -10011.7423)
  ellipse E76 centre (-10075.2788, -10011.5783) end of major axis (-10075.513, -10009.5015) minor radius 0.0445 (-10075.5166, -10009.5697) -> (-10075.4863, -10009.995) ccw
  ellipse E77 centre (-10074.3847, -10011.4775) end of major axis (-10074.6189, -10009.4006) minor radius 0.0445 (-10074.6224, -10009.4715) -> (-10074.5924, -10009.8906) ccw
  ellipse E78 centre (-10060.476, -10009.9089) end of major axis (-10060.3863, -10010.7038) minor radius 0.017 (-10060.4845, -10009.9851) -> (-10060.3936, -10010.678) ccw
  line L94 (-10060.3779, -10010.9136) -> (-10060.4845, -10009.9851)
  ellipse E79 centre (-10059.4825, -10009.7968) end of major axis (-10059.4265, -10010.2937) minor radius 0.0106 (-10059.5392, -10009.3223) -> (-10059.4292, -10010.2861) ccw
  line L95 (-10062.35, -10017.5176) -> (-10062.8067, -10017.4679)
  line L96 (-10060.4543, -10015.4301) -> (-10060.4606, -10016.5807)
  line L97 (-10059.8803, -10016.4222) -> (-10059.8731, -10015.1101)
  line L98 (-10059.8731, -10015.1101) -> (-10060.0464, -10015.004)
  ellipse E80 centre (-10060.05, -10015.6777) end of major axis (-10060.2343, -10014.966) minor radius 0.3717 (-10060.4426, -10015.282) -> (-10060.4543, -10015.4301) ccw
  ellipse E81 centre (-10060.05, -10015.6777) end of major axis (-10060.2343, -10014.966) minor radius 0.3717 (-10060.0464, -10015.004) -> (-10060.0542, -10014.9994) ccw
  ellipse E82 centre (-10059.335, -10016.8242) end of major axis (-10059.2485, -10016.0289) minor radius 0.2736 (-10059.1014, -10016.2094) -> (-10059.1558, -10016.0937) ccw
  line L99 (-10062.35, -10020.5126) -> (-10062.8067, -10020.5623)
  ellipse E83 centre (-10060.0254, -10022.3725) end of major axis (-10059.9322, -10021.6648) minor radius 0.4004 (-10060.4318, -10022.5398) -> (-10059.9924, -10023.0622) ccw
  line L100 (-10060.0639, -10023.0809) -> (-10060.2044, -10023.0961)
  line L101 (-10060.4764, -10021.6089) -> (-10060.4318, -10022.5398)
  line L102 (-10059.9924, -10023.0622) -> (-10059.8183, -10022.9906)
  line L103 (-10059.8183, -10022.9906) -> (-10059.8765, -10021.7728)
  ellipse E84 centre (-10059.335, -10021.3698) end of major axis (-10059.2485, -10022.1651) minor radius 0.2736 (-10059.1558, -10022.1003) -> (-10059.1014, -10021.9846) ccw
  ellipse E85 centre (-10061.4695, -10028.1731) end of major axis (-10061.5591, -10028.968) minor radius 0.017 (-10061.4873, -10028.1788) -> (-10061.5607, -10028.9553) ccw
  line L104 (-10061.4873, -10028.1788) -> (-10061.3802, -10027.2277)
  ellipse E86 centre (-10059.4825, -10028.3972) end of major axis (-10059.5722, -10029.1921) minor radius 0.017 (-10059.4076, -10027.6709) -> (-10059.5711, -10029.1195) ccw
  line L105 (-10061.565, -10026.5852) -> (-10062.0782, -10026.5274)
  ellipse E87 centre (-10075.2788, -10026.6157) end of major axis (-10075.513, -10028.6925) minor radius 0.0445 (-10075.4863, -10028.199) -> (-10075.513, -10028.6925) ccw
  ellipse E88 centre (-10074.3847, -10026.7165) end of major axis (-10074.6189, -10028.7933) minor radius 0.0445 (-10074.5924, -10028.3034) -> (-10074.6224, -10028.7225) ccw
  line L106 (-10060.4938, -10028.2908) -> (-10060.38, -10027.2802)
  ellipse E89 centre (-10060.476, -10028.2851) end of major axis (-10060.3863, -10027.4901) minor radius 0.017 (-10060.3936, -10027.516) -> (-10060.4938, -10028.2908) ccw
  ellipse E90 centre (-10059.4825, -10028.3972) end of major axis (-10059.5386, -10028.894) minor radius 0.0106 (-10059.4277, -10027.9536) -> (-10059.5285, -10028.8459) ccw
  line L107 (-10061.4884, -10025.278) -> (-10061.5512, -10026.2627)
  ellipse E91 centre (-10061.3509, -10025.7361) end of major axis (-10061.5168, -10026.5188) minor radius 0.1207 (-10061.5512, -10026.2627) -> (-10061.2503, -10025.8408) ccw
  line L108 (-10061.2503, -10025.8408) -> (-10060.9018, -10024.3132)
  line L109 (-10060.9018, -10024.3132) -> (-10059.9347, -10024.5181)
  ellipse E92 centre (-10059.4168, -10026.1461) end of major axis (-10059.5827, -10026.9287) minor radius 0.1207 (-10059.5154, -10026.8628) -> (-10059.2158, -10025.4549) ccw
  line L110 (-10061.5089, -10026.5204) -> (-10061.5168, -10026.5188)
  line L111 (-10060.9251, -10024.3459) -> (-10060.9018, -10024.3132)
  line L112 (-10060.9018, -10024.3132) -> (-10064.0916, -10023.6371)
  ellipse E93 centre (-10060.3258, -10024.3799) end of major axis (-10060.8847, -10023.5676) minor radius 0.2359 (-10060.1806, -10024.1763) -> (-10060.7921, -10023.5679) ccw
  line L113 (-10061.1009, -10023.5001) -> (-10067.0102, -10022.2476)
  line L114 (-10060.1806, -10024.1763) -> (-10059.9347, -10024.5181)
  line L115 (-10060.2832, -10026.0457) -> (-10059.9347, -10024.5181)
  line L116 (-10061.4225, -10013.1496) -> (-10061.8569, -10013.1724)
  line L117 (-10061.8361, -10012.3263) -> (-10061.5539, -10012.3114)
  line L118 (-10061.4096, -10013.3948) -> (-10061.4924, -10011.8255)
  ellipse E94 centre (-10061.4926, -10011.7733) end of major axis (-10061.5345, -10010.9744) minor radius 0.0026 (-10061.5345, -10010.9744) -> (-10061.4924, -10011.8255) ccw
  line L119 (-10061.3603, -10013.3922) -> (-10061.4096, -10013.3948)
  ellipse E95 centre (-10059.4953, -10011.6684) end of major axis (-10059.5373, -10010.8695) minor radius 0.0026 (-10059.5102, -10011.3406) -> (-10059.5154, -10011.3312) ccw
  line L120 (-10059.5373, -10010.8695) -> (-10061.5345, -10010.9744)
  line L121 (-10061.5577, -10012.0657) -> (-10061.8535, -10012.0812)